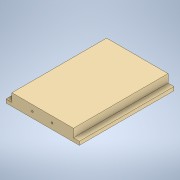
# Autodesk Inventor part: Slider_tatak
Saved by Autodesk Inventor 2021 (Build 250183000, 183)
## iProperties
Created: 2023-04-05
Part Number: Slider_tatak
Material: Generic
Document SubType Name: Modeling
Designer: EF0481
Density: 1 g/cm^3
Appearance: Wheat
Author: EF0481
Autodesk Inventor part; units mm, degrees
ref_plane "YZ Plane" through (0, 0, 0) normal (1, 0, 0) x (0, 1, 0)
ref_plane "XZ Plane" through (0, 0, 0) normal (0, 1, 0) x (-1, 0, 0)
ref_plane "XY Plane" through (0, 0, 0) normal (0, 0, 1) x (1, 0, 0)
sketch "Sketch5" plane through (0, 0, 0) normal (0, 0, 1) x (1, 0, 0)
  line L0 (0, 0) -> (52, 0)
  line L1 (52, 10) -> (0, 10)
  line L2 (0, 0) -> (-5, 0)
  line L3 (-5, 0) -> (-5, 3)
  line L4 (-5, 3) -> (0, 3)
  line L5 (0, 3) -> (0, 10)
  line L6 (52, 0) -> (57, 0)
  line L7 (57, 0) -> (50, 0)
  line L8 (57, 0) -> (57, 0)
  line L9 (50, 0) -> (57, 0)
  line L10 (57, 3) -> (52, 3)
  line L11 (52, 3) -> (52, 10)
  line L12 (57, 3) -> (57, 0)
  dimension "d12" = 52
  dimension "d31" = 3
  dimension "d32" = 5
  dimension "d33" = 5
  dimension "d38" = 3
  dimension "d39" = 10
  dimension "d41" = 5
  constraints: 26 end point, 5 horizontal, 3 perpendicular, 2 parallel, 2 vertical
  measures "d12" distance of L1.end L1.start
  measures "d31" distance of L2.end L3.end
  measures "d32" distance of L0.start L2.end
  measures "d33" distance of L0.end L6.end
  measures "d38" distance of L10.start L7.start
  measures "d39" distance between parallel lines of L0 L1
  measures "d41" distance of L10.start L10.end
extrude "Extrusion2" add sketch "Sketch5" against normal blind 80
sketch "Sketch6" plane through (0, 0, 0) normal (0, 0, 1) x (1, 0, 0)
  circle A0 centre (17.3, 5) radius 0.75
  line L0 (52, 10) -> (0, 10) projected
  line L1 (0, 10) -> (0, 0) projected
  line L2 (0, 10) -> (52, 10) projected
  line L3 (57, 0) -> (0, 0) projected
  circle A1 centre (33.98, 5) radius 0.75
  point P0 (50, 0)
  point P1 (55, 0)
  dimension "d16" = 1.5
  dimension "d17" = 5
  dimension "d19" = 17.3
  dimension "d27" = 16.68
  dimension "d40" = 1.5
  constraints: 2 centre point
  measures "d16" diameter of A0
  measures "d17" distance from line of L0 A0.centre
  measures "d19" distance from line of L1 A0.centre
  measures "d27" distance of A0.centre A1.centre
  measures "d40" diameter of A1
hole "Hole1" at (33.98, 5, 0) at (17.3, 5, 0) direction (0, 0, -1) diameter 1.4249 depth 8.692 thread size "1-64 UNC" class "2B" standard "ANSI Unified Screw Threads"
body "Solid2"
